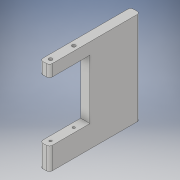
# Autodesk Inventor part: GripperPlate
Saved by Autodesk Inventor 2019 (Build 230136000, 136)
## iProperties
Created: 2019-10-02
Part Number: GripperPlate
Material: Generic
Document SubType Name: Modeling
Designer: james
Density: 1 g/cm^3
Appearance: Default
Mass: 4.85187 g
Surface Area: 34.9632 cm^2
Volume: 4.85187 cm^3
Author: james
Autodesk Inventor part; units mm, degrees
ref_plane "YZ Plane" through (0, 0, 0) normal (1, 0, 0) x (0, 1, 0)
ref_plane "XZ Plane" through (0, 0, 0) normal (0, 1, 0) x (-1, 0, 0)
ref_plane "XY Plane" through (0, 0, 0) normal (0, 0, 1) x (1, 0, 0)
sketch "Sketch1" plane through (0, 0, 0) normal (0, 1, 0) x (-1, 0, 0)
  line L0 (-1.44, 25.5171) -> (-11.6, 25.5171)
  line L1 (-11.6, 25.5171) -> (-11.6, -73.5429)
  line L2 (-11.6, -73.5429) -> (-1.44, -73.5429)
  line L3 (-1.44, -73.5429) -> (-1.44, 25.5171)
  point P0 (0, 0)
  dimension "d0" = 99.06
  dimension "d1" = 10.16
  constraints: 8 end point, 2 parallel, 1 horizontal, 1 perpendicular
  measures "d0" distance of L2.end L0.start
  measures "d1" distance between parallel lines of L1 L3
extrude "Extrusion1" add sketch "Sketch1" along normal blind 101.6
sketch "Sketch2" plane through (0, 101.6, 0) normal (0, 1, 0) x (1, 0, 0)
  line L0 (1.44, -25.5171) -> (11.6, -25.5171) projected
  point P0 (0, 0)
  point P1 (6.5886, -19.1671)
  point P2 (6.5886, 6.2329)
  dimension "d4" = 0
  dimension "d5" = 6.35
  dimension "d6" = 25.4
  measures "d4" horizontal distance of point (6.589, -19.167) point (6.589, 6.233)
  measures "d5" distance from line of L0 point (6.589, -19.167)
  measures "d6" distance of point (6.589, -19.167) point (6.589, 6.233)
hole "Hole1" at (6.5886, 101.6, 19.1671) at (6.5886, 101.6, -6.2329) direction (0, -1, 0) diameter 2.6416 end through all thread size "6-32 UNC" class "2B" standard "ANSI Unified Screw Threads"
sketch "Sketch3" plane through (11.6, 0, 25.5171) normal (1, 0, 0) x (0, 0, -1)
  line L0 (12.7, 88.9) -> (-33.0221, 88.9)
  line L1 (-33.0221, 88.9) -> (-33.0221, 24.13)
  line L2 (-33.0221, 24.13) -> (12.7, 24.13)
  line L3 (12.7, 24.13) -> (12.7, 88.9)
  line L4 (0, 101.6) -> (99.06, 101.6) projected
  line L5 (0, 0) -> (0, 101.6) projected
  point P0 (25.5171, 0)
  dimension "d15" = 12.7
  dimension "d16" = 64.77
  dimension "d19" = 12.7
  constraints: 8 end point, 2 parallel, 1 horizontal, 1 perpendicular
  measures "d15" distance between parallel lines of L4 L0
  measures "d16" distance of L0.end L1.end
  measures "d19" distance between parallel lines of L3 L5
extrude "Extrusion2" cut sketch "Sketch3" against normal blind 25.4
sketch "Sketch4" plane through (11.6, 0, 25.5171) normal (1, 0, 0) x (0, 0, -1)
  line L0 (12.7, 24.13) -> (44.45, 24.13)
  line L1 (44.45, 24.13) -> (44.45, 88.9)
  line L2 (44.45, 88.9) -> (12.7, 88.9)
  line L3 (12.7, 88.9) -> (12.7, 24.13)
  line L4 (0, 88.9) -> (12.7, 88.9) projected
  line L5 (12.7, 24.13) -> (0, 24.13) projected
  line L6 (12.7, 88.9) -> (12.7, 24.13) projected
  point P0 (25.5171, 0)
  dimension "d20" = 31.75
  dimension "d21" = 0
  dimension "d22" = 0
  dimension "d23" = 0
  constraints: 8 end point, 2 parallel, 1 horizontal, 1 perpendicular
  measures "d20" distance between parallel lines of L3 L1
  measures "d21" distance between parallel lines of L4 L2
  measures "d22" distance between parallel lines of L5 L0
  measures "d23" distance between parallel lines of L6 L3
extrude "Extrusion3" cut sketch "Sketch4" against normal blind 25.4
sketch "Sketch5" plane through (0, 101.6, 0) normal (0, 1, 0) x (1, 0, 0)
  circle A0 centre (6.5886, 6.2329) radius 1.3208 projected
  circle A1 centre (6.5886, -19.1671) radius 1.3208 projected
  point P0 (0, 0)
  constraints: 2 coincident
hole "Hole2" at (6.5886, 101.6, 19.1671) at (6.5886, 101.6, -6.2329) direction (0, -1, 0) diameter 3.81 depth 15.24 tip angle 118.188 clearance for "Flat Head Machine Screw (82)" size "#6" standard "Ansi Unified Screw Threads"
fillet "Fillet1" radius 3.175 1 edges at (11.6, 95.25, 25.5171)
fillet "Fillet2" radius 3.175 5 edges at (11.6, 12.065, 25.5171) (1.44, 12.065, 25.5171) (1.44, 95.25, 25.5171) (11.6, 50.8, -73.5429) (1.44, 50.8, -73.5429)
body "Solid1"
